Autodesk Inventor part; units mm, degrees
(part 2 of 2)
  line L145 (-20.1977, 92.6589) -> (-20.1977, 93.0121)
  spline S95 degree 2 poles (-22.4528, 92.0439) (-22.4528, 92.2637) (-22.312, 92.6391) (-22.1836, 92.7774) knots 0 0 0 1 2 2 2
  spline S96 degree 2 poles (-22.1836, 92.7774) (-22.0551, 92.9158) (-21.6723, 93.0763) (-21.4351, 93.0763) knots 0 0 0 1 2 2 2
  spline S97 degree 2 poles (-21.4351, 93.0763) (-21.2178, 93.0763) (-20.7929, 92.98) (-20.6373, 92.9034) knots 0 0 0 1 2 2 2
  line L146 (-20.6373, 92.9034) -> (-20.6373, 92.4712)
  line L147 (-20.6373, 92.4712) -> (-20.667, 92.4712)
  spline S98 degree 2 poles (-20.667, 92.4712) (-20.7139, 92.5057) (-20.8893, 92.5947) (-20.9955, 92.6342) knots 0 0 0 1 2 2 2
  spline S99 degree 2 poles (-20.9955, 92.6342) (-21.1165, 92.6762) (-21.3166, 92.7231) (-21.4426, 92.7231) knots 0 0 0 1 2 2 2
  spline S100 degree 2 poles (-21.4426, 92.7231) (-21.5661, 92.7231) (-21.7982, 92.6342) (-21.8822, 92.5379) knots 0 0 0 1 2 2 2
  spline S101 degree 2 poles (-21.8822, 92.5379) (-21.9588, 92.4465) (-22.0378, 92.2044) (-22.0378, 92.0414) knots 0 0 0 1 2 2 2
  spline S102 degree 2 poles (-22.0378, 92.0414) (-22.0378, 91.8784) (-21.9489, 91.6709) (-21.8649, 91.6017) knots 0 0 0 1 2 2 2
  spline S103 degree 2 poles (-21.8649, 91.6017) (-21.7785, 91.5251) (-21.5216, 91.4609) (-21.366, 91.4609) knots 0 0 0 1 2 2 2
  spline S104 degree 2 poles (-21.366, 91.4609) (-21.198, 91.4609) (-20.8646, 91.5128) (-20.7633, 91.535) knots 0 0 0 1 2 2 2
  line L148 (-20.7633, 91.535) -> (-20.7633, 89.9641)
  line L149 (-20.7633, 89.9641) -> (-22.4355, 89.9641)
  line L150 (-22.4355, 89.9641) -> (-22.4355, 90.3222)
  line L151 (-22.4355, 90.3222) -> (-21.156, 90.3222)
  line L152 (-21.156, 90.3222) -> (-21.156, 91.1349)
  spline S105 degree 2 poles (-21.156, 91.1349) (-21.2301, 91.125) (-21.3734, 91.1176) (-21.4327, 91.1176) knots 0 0 0 1 2 2 2
  spline S106 degree 2 poles (-21.4327, 91.1176) (-21.6673, 91.1176) (-21.9909, 91.1942) (-22.1391, 91.3078) knots 0 0 0 1 2 2 2
  spline S107 degree 2 poles (-22.1391, 91.3078) (-22.2898, 91.4214) (-22.4528, 91.7672) (-22.4528, 92.0439) knots 0 0 0 1 2 2 2
  point P0 (-47.5, 53.2457)
  constraints: 2 other
extrude "Extrusion47" add sketch "Sketch58" along normal blind 1
sketch "Sketch59" plane through (69.5, 80.5, 0) normal (0, 0, -1) x (-1, 0, 0)
  line L0 (124.232, -148.2248) -> (124.232, -65.5994) projected
  line L1 (124.232, -131.7625) -> (22.225, -131.7625)
  line L2 (22.225, -144.4625) -> (124.232, -144.4625)
  line L3 (124.232, -144.4625) -> (124.232, -131.7625)
  line L4 (22.225, -144.4625) -> (19.05, -144.4625)
  line L5 (19.05, -144.4625) -> (19.05, -131.7625)
  line L6 (19.05, -131.7625) -> (22.225, -131.7625)
  point P0 (69.5, -80.5)
  point P1 (22.225, -131.7625)
  constraints: 12 end point, 2 horizontal, 2 parallel, 1 perpendicular, 1 point on line
extrude "Extrusion48" add sketch "Sketch59" against normal blind 1
extrude "Extrusion49" cut sketch "Sketch57" against normal blind 3 contours A0 | A2 | A4 | A5 | A7 | A9
body "Solid1"
